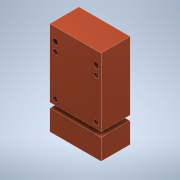
# Autodesk Inventor part: NF TC-02
Saved by Autodesk Inventor 2021 (Build 250183000, 183)
## iProperties
Created: 2023-01-29
Part Number: NF TC-02
Material: Cobre, aleado
Document SubType Name: Modeling
Designer: Diego.labarca
Density: 8.92 g/cm^3
Appearance: Cobre - Satinado
Author: Diego.labarca
Autodesk Inventor part; units mm, degrees
ref_plane "YZ Plane" through (0, 0, 0) normal (1, 0, 0) x (0, 1, 0)
ref_plane "XZ Plane" through (0, 0, 0) normal (0, 1, 0) x (-1, 0, 0)
ref_plane "XY Plane" through (0, 0, 0) normal (0, 0, 1) x (1, 0, 0)
sketch "Boceto1" plane through (0, 0, 0) normal (0, 0, 1) x (1, 0, 0)
  line L0 (-15, 20) -> (15, 20)
  line L1 (15, 20) -> (15, -20)
  line L2 (15, -20) -> (-15, -20)
  line L3 (-15, -20) -> (-15, 20)
  line L4 (5.2741, 0) -> (0, 0)
  line L5 (0, 0) -> (0, 2.4047)
  dimension "d0" = 30
  dimension "d1" = 40
  constraints: 12 end point, 2 horizontal, 2 parallel, 2 perpendicular, 2 other
  measures "d0" distance of L1.end L2.end
  measures "d1" distance of L0.end L1.end
extrude "Extrusión1" add sketch "Boceto1" along normal blind 17
sketch "Boceto2" plane through (0, 0, 17) normal (0, 0, 1) x (1, 0, 0)
  circle A0 centre (12, -17) radius 1.5
  line L0 (15, -20) -> (15, 20) projected
  line L1 (-15, -20) -> (15, -20) projected
  circle A1 centre (12, 7) radius 1.5
  circle A2 centre (12, 12.1331) radius 1.75
  point P0 (0, 0)
  dimension "d4" = 3
  dimension "d5" = 3
  dimension "d6" = 3
  dimension "d7" = 3
  dimension "d8" = 3
  dimension "d9" = 24
  dimension "d10" = 3.5
  dimension "d11" = 3
  constraints: 3 centre point
  measures "d4" diameter of A0
  measures "d5" distance from line of L0 A0.centre
  measures "d6" distance from line of A0.centre L1
  measures "d7" diameter of A1
  measures "d8" distance from line of A1.centre L0
  measures "d9" distance of A0.centre A1.centre
  measures "d10" diameter of A2
  measures "d11" distance from line of L0 A2.centre
extrude "Extrusión2" cut sketch "Boceto2" against normal through all
mirror "Simetría1" about plane through (0, 0, 0) normal (1, 0, 0) of "Extrusión2"
sketch "Boceto3" plane through (0, 0, 17) normal (0, 0, 1) x (1, 0, 0)
  line L0 (-15, -23) -> (15, -23)
  line L1 (15, -23) -> (15, -35)
  line L2 (15, -35) -> (-15, -35)
  line L3 (-15, -35) -> (-15, -23)
  line L4 (-15, -20) -> (15, -20) projected
  point P0 (0, 0)
  dimension "d14" = 12
  dimension "d22" = 3
  constraints: 8 end point, 2 parallel, 1 horizontal, 1 perpendicular
  measures "d14" distance of L0.end L1.end
  measures "d22" distance between parallel lines of L0 L4
extrude "Extrusión3" add sketch "Boceto3" against normal up to surface (17 mm away)
sketch "Boceto4" plane through (0, 0, 0) normal (1, 0, 0) x (0, 1, 0)
  line L0 (-38.5, 5.5) -> (-35, 5.5)
  line L1 (-35, 17) -> (-35, 0) projected
  line L2 (-23, 0) -> (-35, 0) projected
  line L3 (-23, 17) -> (-23, 0) projected
  line L4 (-23, 5.5) -> (-20, 5.5)
  line L5 (-20, 0) -> (-20, 17) projected
  line L6 (-41, 8.5) -> (-20, 8.5)
  line L7 (-41, 8.5) -> (-41, 8)
  line L8 (-41, 8) -> (-38.5, 5.5)
  point P0 (0, 0)
  point P1 (-35, 8.5)
  point P2 (-23, 8.5)
  dimension "d18" = 6
  dimension "d19" = 3
  dimension "d20" = 8.5
  dimension "d23" = 0.5
  dimension "d24" = 135
  constraints: 10 end point, 3 point on line, 2 horizontal, 1 midpoint, 1 vertical
  measures "d18" distance from line of L6.start L1
  measures "d19" distance from line of L6.start L0
  measures "d20" distance from line of L6.start L2
  measures "d23" distance of L6.start L7.end
  measures "d24" angle of L7 L8
revolve "Revolución1" add sketch "Boceto4" angle 360 about axis through (0, -41, 8.5) along (0, 1, 0) contours L8 L7 L6 L1 L0 | L6 L5 L4 L3
equation "\"d7\" = d4"
equation "\"d8\" = d5"
equation "\"d11\" = d8"
